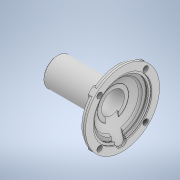
# Autodesk Inventor part: 73. Крышка подшипника
Saved by Autodesk Inventor 2021 (Build 250183000, 183)
## iProperties
Created: 2021-03-25
Part Number: 73. Крышка подшипника
Material: Типовые
Document SubType Name: Modeling
Designer: Данил
Density: 1 g/cm^3
Appearance: По умолчанию
Author: Данил
Autodesk Inventor part; units mm, degrees
ref_plane "YZ Plane" through (0, 0, 0) normal (1, 0, 0) x (0, 1, 0)
ref_plane "XZ Plane" through (0, 0, 0) normal (0, 1, 0) x (-1, 0, 0)
ref_plane "XY Plane" through (0, 0, 0) normal (0, 0, 1) x (1, 0, 0)
sketch "Эскиз1" plane through (0, 0, 0) normal (0, 0, 1) x (1, 0, 0)
  line L0 (-51, 0) -> (51, 0)
  line L1 (-51, -21.2) -> (-51, -20)
  line L2 (-51, -20) -> (-47.5359, -18)
  line L3 (-50.2, -22) -> (27.5, -22)
  line L4 (-47.5359, -18) -> (17, -18)
  line L5 (-50.2, -22) -> (-51, -21.2)
  line L6 (17, -18) -> (36, -18)
  line L7 (29, -23.5) -> (29, -24)
  line L8 (29, -24) -> (31, -24)
  line L9 (32.4266, -25.0365) -> (41.6777, -53.5086)
  arc A0 (29, -23.5) -> (27.5, -22) centre (27.5, -23.5) ccw
  arc A1 (32.4266, -25.0365) -> (31, -24) centre (31, -25.5) ccw
  line L10 (47.8596, -58) -> (51, -58)
  arc A2 (41.6777, -53.5086) -> (47.8596, -58) centre (47.8596, -51.5) ccw
  line L11 (51, -58) -> (51, -46)
  line L12 (36, -24.1428) -> (36, -18)
  line L13 (36.0865, -24.5495) -> (40.7958, -35.1269)
  line L14 (44.45, -37.5) -> (44.45, -37.5)
  line L15 (44.45, -37.5) -> (44.45, -42.75)
  arc A3 (36, -24.1428) -> (36.0865, -24.5495) centre (37, -24.1428) ccw
  arc A4 (40.7958, -35.1269) -> (44.45, -37.5) centre (44.45, -33.5) ccw
  line L16 (44.95, -43.25) -> (45.95, -43.25)
  line L17 (46.45, -42.75) -> (46.45, -42.5)
  line L18 (46.45, -42.5) -> (49, -42.5)
  arc A5 (44.45, -42.75) -> (44.95, -43.25) centre (44.95, -42.75) ccw
  arc A6 (45.95, -43.25) -> (46.45, -42.75) centre (45.95, -42.75) ccw
  line L19 (49, -42.5) -> (49, -45.8)
  line L20 (49.2, -46) -> (51, -46)
  arc A7 (49, -45.8) -> (49.2, -46) centre (49.2, -45.8) ccw
  point P0 (0, 0)
  point P1 (0, 0)
  point P2 (-51, -22)
  point P3 (36, -24.3554)
  point P4 (44.45, -37.5)
  dimension "d0" = 102
  dimension "d1" = 36
  dimension "d2" = 44
  dimension "d3" = 40
  dimension "d4" = 0.8
  dimension "d5" = 45
  dimension "d6" = 30
  dimension "d7" = 68
  dimension "d8" = 1.5
  dimension "d9" = 18
  dimension "d10" = 116
  dimension "d11" = 48
  dimension "d12" = 6.5
  dimension "d14" = 15
  dimension "d15" = 20
  dimension "d18" = 2
  dimension "d20" = 1
  dimension "d21" = 4
  dimension "d22" = 24
  dimension "d23" = 2
  dimension "d24" = 0.75
  dimension "d25" = 0.5
  dimension "d26" = 0.2
  dimension "d27" = 92
  dimension "d28" = 85
  dimension "d29" = 75
  dimension "d30" = 2
  dimension "d31" = 4.55
  constraints: 42 end point, 16 point on circle, 16 tangent, 8 centre point, 7 horizontal, 5 perpendicular, 5 vertical, 4 point on line, 3 vertical alignment, 2 equal radius, 1 coincident, 1 midpoint
  measures "d0" distance of L0.start L0.end
  measures "d1" diameter of L4 L0
  measures "d2" diameter of L3 L0
  measures "d3" diameter of L1.end L0
  measures "d4" distance of L3.start point (-51, -22)
  measures "d5" angle of L3 L5
  measures "d6" angle of L3 L2
  measures "d7" horizontal distance of L0.start L4.end
  measures "d8" radius of A0
  measures "d9" angle of L7 L9
  measures "d10" diameter of L10 L0
  measures "d11" diameter of L8 L0
  measures "d12" radius of A2
  measures "d14" distance from line of L0.end L12
  measures "d15" horizontal distance of L0.end L8.end
  measures "d18" distance of L7.end L8.end
  measures "d20" radius of A3
  measures "d21" radius of A4
  measures "d22" angle of L12 L13
  measures "d23" distance between parallel lines of L15 L17
  measures "d24" distance between parallel lines of L16 L18
  measures "d25" radius of A5
  measures "d26" radius of A7
  measures "d27" diameter of L11.end L0
  measures "d28" diameter of L18 L0
  measures "d29" diameter of L14 L0
  measures "d30" distance from line of L19 L0.end
  measures "d31" distance between parallel lines of L15 L19
revolve "Вращение1" add sketch "Эскиз1" angle 360 about axis through (-51, 0, 0) along (1, 0, 0)
sketch "Эскиз2" plane through (51, 0, 0) normal (1, 0, 0) x (0, 0, -1)
  circle A0 centre (0, 0) radius 58 projected
  line L0 (0, 0) -> (0, -58) construction
  circle A1 centre (0, 0) radius 58 projected
  line L1 (0, 0) -> (-5.055, -57.7793) construction
  arc A2 (-10.3695, -44.6708) -> (-4.4449, -50.8059) centre (-3.8784, -44.3307) ccw
  arc A3 (0, -51) -> (6.4753, -45.0665) centre (0, -44.5) ccw
  circle A4 centre (0, 0) radius 46 projected
  circle A5 centre (0, 0) radius 51
  line L2 (-10.3695, -44.6708) -> (-12.7106, 0)
  line L3 (6.4753, -45.0665) -> (10.4181, 0)
  circle A6 centre (0, 0) radius 24 projected
  line L4 (-12.7106, 0) -> (10.4181, 0)
  point P0 (0, 0)
  dimension "d32" = 5
  dimension "d33" = 6.5
  dimension "d34" = 102
  dimension "d35" = 5
  dimension "d36" = 8
  constraints: 10 end point, 8 point on circle, 4 point on line, 4 tangent, 3 centre point, 2 horizontal alignment, 1 coincident, 1 equal radius, 1 horizontal, 1 vertical
  measures "d32" angle of L0 L1
  measures "d33" radius of A3
  measures "d34" diameter of A5
  measures "d35" angle of L3 L0
  measures "d36" angle of L2 L1
extrude "Выдавливание1" cut sketch "Эскиз2" against normal up to surface contours L2 A6 L3 A3 A4 A2 | A4 A3 A5 A2 | L2 L4 L3 A6 round surface about axis through (38.4411, 0, 0) along (-1, 0, 0) radius 29.8382 half angle -66 far side no picked at (-5.6401, -38.1184) picked at (-1.8296, -47.573) picked at (-1.3436, -7.979)
ref_plane "РабПлоскость1" through (41.5, 0, 0) normal (1, 0, 0) x (0, 0, -1)
sketch "Эскиз3" plane through (41.5, 0, 0) normal (1, 0, 0) x (0, 0, -1)
  circle A0 centre (0, 0) radius 51 construction
  circle A1 centre (-36.0624, 36.0624) radius 8.5
  line L0 (0, 0) -> (0, 51) construction
  line L1 (0, 0) -> (-36.0624, 36.0624) construction
  circle A2 centre (-36.0624, 36.0624) radius 4.25
  circle A3 centre (36.0624, 36.0624) radius 8.5
  circle A4 centre (36.0624, 36.0624) radius 4.25
  circle A5 centre (36.0624, -36.0624) radius 8.5
  circle A6 centre (36.0624, -36.0624) radius 4.25
  circle A7 centre (-36.0624, -36.0624) radius 8.5
  circle A8 centre (-36.0624, -36.0624) radius 4.25
  circle A9 centre (0, 0) radius 58 projected
  circle A10 centre (0, 0) radius 53.5086 projected
  point P0 (-31.5146, -43.2435)
  point P1 (-35.2713, -40.2382)
  point P2 (-40.2382, -35.2713)
  point P3 (-43.2435, -31.5146)
  point P4 (-44.4835, -37.2186)
  point P5 (-37.2186, -44.4835)
  dimension "d40" = 102
  dimension "d41" = 17
  dimension "d42" = 45
  dimension "d43" = 8.5
  dimension "d46" = 360
  constraints: 9 centre point, 5 coincident, 4 end point, 2 point on circle, 1 vertical, 17 other
  measures "d40" diameter of A0
  measures "d41" diameter of A1
  measures "d42" angle of L1 L0
  measures "d43" diameter of A2
extrude "Выдавливание2" cut sketch "Эскиз3" against normal through all both and the other way through all contours A10 A2 | A2 A10 | A10 A4 | A4 A10 | A10 A8 | A8 A10 | A10 A6 | A6 A10
extrude "Выдавливание3" cut sketch "Эскиз3" against normal through all contours A1 A10 A2 | A10 A2 A1 A9 | A9 A1 | A10 A4 A3 | A3 A9 A10 A4 | A10 A8 A7 A9 | A7 A10 A8 | A3 A9 | A9 A7 | A10 A6 A5 | A5 A9 A10 A6 | A9 A5
extrude "Выдавливание4" add sketch "Эскиз3" along normal blind 9.5 contours A10 A8 A7 A9
pattern_circular "Круговой массив1" count 4 over 360 about axis through (-11.35, 0, 0) along (-1, 0, 0) of "Выдавливание4"
extrude "Выдавливание5" add sketch "Эскиз3" along normal blind 1 contours A7 A10 A8
pattern_circular "Круговой массив2" count 4 over 360 about axis through (-11.35, 0, 0) along (-1, 0, 0) of "Выдавливание5"
sketch "Эскиз4" plane through (41.5, 0, 0) normal (-1, 0, 0) x (0, 0, 1)
  circle A0 centre (0, 0) radius 54
  circle A1 centre (0, 0) radius 58
  arc A2 (-44.4835, 37.2186) -> (-42.916, 31.0346) centre (-36.0624, 36.0624) ccw projected
  arc A3 (-31.0346, 42.916) -> (-37.2186, 44.4835) centre (-36.0624, 36.0624) ccw projected
  arc A4 (37.2186, 44.4835) -> (31.0346, 42.916) centre (36.0624, 36.0624) ccw projected
  arc A5 (42.916, 31.0346) -> (44.4835, 37.2186) centre (36.0624, 36.0624) ccw projected
  arc A6 (44.4835, -37.2186) -> (42.916, -31.0346) centre (36.0624, -36.0624) ccw projected
  arc A7 (31.0346, -42.916) -> (37.2186, -44.4835) centre (36.0624, -36.0624) ccw projected
  arc A8 (-37.2186, -44.4835) -> (-31.0346, -42.916) centre (-36.0624, -36.0624) ccw projected
  arc A9 (-42.916, -31.0346) -> (-44.4835, -37.2186) centre (-36.0624, -36.0624) ccw projected
  point P0 (-43.5153, -31.9753)
  point P1 (-43.5153, 31.9753)
  point P2 (-31.9753, -43.5153)
  point P3 (31.9753, -43.5153)
  point P4 (31.9753, 43.5153)
  point P5 (-31.9753, 43.5153)
  point P6 (43.5153, -31.9753)
  point P7 (43.5153, 31.9753)
  dimension "d63" = 116
  dimension "d62" = 108
  constraints: 2 coincident, 1 centre point, 2 other
  measures "d62" diameter of A0
extrude "Выдавливание6" cut sketch "Эскиз4" against normal blind 1.5 contours A0 A5 A1 A6 | A0 A3 A1 A4 | A7 A1 A8 A0 | A0 A9 A1 A2
chamfer "Фаска1" distance 1 angle 15 1 edges at (41.5, 41.0122, 41.0122) measured on face at (41.5, 40.6586, 40.6586)
chamfer "Фаска2" distance 1 angle 15 1 edges at (41.5, 41.0122, -41.0122) measured on face at (41.5, 40.6586, -40.6586)
chamfer "Фаска3" distance 1 angle 15 1 edges at (41.5, -41.0122, -41.0122) measured on face at (41.5, -40.6586, -40.6586)
chamfer "Фаска4" distance 1 angle 15 1 edges at (41.5, -41.0122, 41.0122) measured on face at (41.5, -40.6586, 40.6586)
